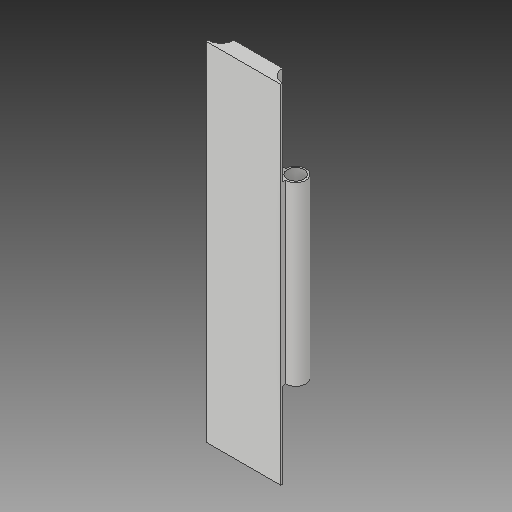
# Autodesk Inventor part: innerFrontPlate
Saved by Autodesk Inventor 2019 (Build 230136000, 136)
## iProperties
Created: 2018-07-23
Part Number: innerFrontPlate
Material: Generic
Document SubType Name: Modeling
Designer: Ge Shi
Density: 1 g/cm^3
Appearance: Default
Author: Ge Shi
Autodesk Inventor part; units mm, degrees
ref_plane "YZ Plane" through (0, 0, 0) normal (1, 0, 0) x (0, 1, 0)
ref_plane "XZ Plane" through (0, 0, 0) normal (0, 1, 0) x (-1, 0, 0)
ref_plane "XY Plane" through (0, 0, 0) normal (0, 0, 1) x (1, 0, 0)
sketch "Sketch1" plane through (0, 0, 0) normal (0, 0, 1) x (1, 0, 0)
  line L0 (10, -46.5) -> (-10, -46.5)
  line L1 (-10, -46.5) -> (-10, 46.5)
  line L2 (-10, 46.5) -> (10, 46.5)
  line L3 (10, 46.5) -> (10, -46.5)
  line L4 (10, -46.5) -> (-10, 46.5) construction
  line L5 (-10, -46.5) -> (10, 46.5) construction
  point P0 (0, 0)
  dimension "d0" = 20
  dimension "d1" = 93
  constraints: 12 end point, 2 midpoint, 2 parallel, 1 horizontal, 1 perpendicular
  measures "d0" distance of L1.end L2.end
  measures "d1" distance of L0.end L1.end
extrude "Extrusion1" add sketch "Sketch1" along normal blind 4
ref_plane "Work Plane1" through (-10, 0, 0) normal (0, 1, 0) x (1, 0, 0)
sketch "Sketch2" plane through (-10, 0, 0) normal (0, 1, 0) x (1, 0, 0)
  circle A0 centre (0, 0) radius 2.25
  circle A1 centre (0, 0) radius 2.75
  circle A2 centre (0, 0) radius 3.5
  circle A3 centre (20, 0) radius 2.25
  circle A4 centre (20, 0) radius 2.75
  circle A5 centre (20, 0) radius 3.5
  point P0 (10, 0)
  dimension "d4" = 4.5
  dimension "d5" = 5.5
  dimension "d6" = 7
  dimension "d7" = 4.5
  dimension "d8" = 5.5
  dimension "d9" = 7
  constraints: 6 centre point, 4 coincident
  measures "d4" diameter of A0
  measures "d5" diameter of A1
  measures "d6" diameter of A2
  measures "d7" diameter of A3
  measures "d8" diameter of A4
  measures "d9" diameter of A5
extrude "Extrusion2" cut sketch "Sketch2" along normal mid plane 93 contours A0 | A1 | A3 | A4
extrude "Extrusion3" add sketch "Sketch2" along normal mid plane 47.25 contours A1 | A4
extrude "Extrusion4" cut sketch "Sketch2" against normal blind 50 from surface at -23.625 contours A2
extrude "Extrusion5" cut sketch "Sketch2" against normal blind 50 from surface at -23.625 contours A5
extrude "Extrusion6" cut sketch "Sketch2" along normal blind 50 from surface at 23.625 contours A2
extrude "Extrusion7" cut sketch "Sketch2" along normal blind 50 from surface at 23.625 contours A5
equation "\"d0\" = folderLength"
equation "\"d1\" = -hingeShaftHolder + height - clearance"
equation "\"d2\" = thick"
equation "\"d4\" = hingeShaft + clearance"
equation "\"d5\" = hingeShaftHolder"
equation "\"d6\" = hingeShaftHolder + clearance"
equation "\"d7\" = hingeShaft + clearance"
equation "\"d8\" = hingeShaftHolder"
equation "\"d9\" = hingeShaftHolder + clearance"
equation "\"d10\" = -hingeShaftHolder + height - clearance"
equation "\"d14\" = 0.5 * height"
equation "\"d16\" = 0.5 * height"
equation "\"d18\" = 0.5 * height"
equation "\"d20\" = 0.5 * height"
equation "\"folderLength\" = 20"
equation "\"hingeShaftHolder\" = 5.5"
equation "\"height\" = 100"
equation "\"clearance\" = 1.5"
equation "\"thick\" = 4"
equation "\"hingeShaft\" = 3"
body "Solid1"
